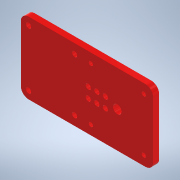
# Autodesk Inventor part: housingBack
Saved by Autodesk Inventor 2020 (Build 240168000, 168)
## iProperties
Created: 2020-02-03
Part Number: housingBack
Material: ABS Plastic
Document SubType Name: Modeling
Designer: Felix
Density: 1.06 g/cm^3
Appearance: Smooth - Red
Author: Felix
Autodesk Inventor part; units mm, degrees
ref_plane "YZ Plane" through (0, 0, 0) normal (1, 0, 0) x (0, 1, 0)
ref_plane "XZ Plane" through (0, 0, 0) normal (0, 1, 0) x (-1, 0, 0)
ref_plane "XY Plane" through (0, 0, 0) normal (0, 0, 1) x (1, 0, 0)
sketch "Sketch1" plane through (0, 0, 0) normal (0, 0, 1) x (1, 0, 0)
  line L0 (21.5, 21) -> (-21.5, 21) projected
  arc A0 (-21.5, 21) -> (-26, 16.5) centre (-21.5, 16.5) ccw construction
  line L1 (-26, 16.5) -> (-26, -16.5) construction
  arc A1 (-26, -16.5) -> (-21.5, -21) centre (-21.5, -16.5) ccw construction
  line L2 (-21.5, -21) -> (21.5, -21) projected
  arc A2 (21.5, -21) -> (26, -16.5) centre (21.5, -16.5) ccw construction
  line L3 (26, -16.5) -> (26, 16.5) construction
  arc A3 (26, 16.5) -> (21.5, 21) centre (21.5, 16.5) ccw construction
  circle A4 centre (5, 0) radius 2.5 projected
  circle A5 centre (-20, 15.5) radius 1.5 projected
  circle A6 centre (-10.5, -15.5) radius 1.2295 projected
  circle A7 centre (-10.5, 15.5) radius 1.2295 projected
  circle A8 centre (-2, 3) radius 1.5 projected
  circle A9 centre (-2, -3) radius 1.5 projected
  circle A10 centre (-7, 3) radius 1.5 projected
  circle A11 centre (-7, -3) radius 1.5 projected
  circle A12 centre (-12, 3) radius 1.5 projected
  circle A13 centre (-12, -3) radius 1.5 projected
  circle A14 centre (-20, -15.5) radius 1.5 projected
  circle A15 centre (20.5, -15.5) radius 1.2295 projected
  circle A16 centre (20.5, 15.5) radius 1.2295 projected
  line L4 (-21.5, 21) -> (-47, 21)
  line L5 (-51.5, 16.5) -> (-51.5, -16.5)
  line L6 (-47, -21) -> (-21.5, -21)
  arc A17 (-47, 21) -> (-51.5, 16.5) centre (-47, 16.5) ccw
  arc A18 (-51.5, -16.5) -> (-47, -21) centre (-47, -16.5) ccw
  circle A19 centre (-47, -16.5) radius 1.5
  circle A20 centre (-47, 16.5) radius 1.5
  line L7 (21.5, 21) -> (32, 21)
  line L8 (36.5, 16.5) -> (36.5, -16.5)
  line L9 (32, -21) -> (21.5, -21)
  arc A21 (36.5, 16.5) -> (32, 21) centre (32, 16.5) ccw
  arc A22 (32, -21) -> (36.5, -16.5) centre (32, -16.5) ccw
  circle A23 centre (32, 16.5) radius 1.5
  circle A24 centre (32, -16.5) radius 1.5
  point P0 (0, 0)
  point P1 (-51.5, 21)
  point P2 (36.5, 21)
  dimension "d0" = 30
  dimension "d1" = 4.5
  dimension "d2" = 3
  dimension "d3" = 3
  dimension "d13" = 15
  dimension "d14" = 4.5
  dimension "d15" = 3
  dimension "d16" = 3
  constraints: 12 end point, 9 point on circle, 8 centre point, 8 tangent, 5 point on line, 4 coincident, 3 perpendicular, 2 collinear, 2 equal radius, 1 horizontal
  measures "d0" distance of L0.end point (-51.5, 21)
  measures "d1" radius of A17
  measures "d2" diameter of A19
  measures "d3" diameter of A20
  measures "d13" distance of L7.start point (36.5, 21)
  measures "d14" radius of A21
  measures "d15" diameter of A23
  measures "d16" diameter of A24
extrude "Extrusion1" add sketch "Sketch1" along normal blind 3.5
ref_plane "Work Plane1" through (0, 0, 10.75) normal (0, 0, -1) x (-1, 0, 0)
sketch "Sketch2" plane through (0, 0, 0) normal (0, 0, -1) x (-1, 0, 0)
  circle A0 centre (-20.5, 15.5) radius 1.2295 projected
  circle A1 centre (-20.5, 15.5) radius 3
  circle A2 centre (10.5, 15.5) radius 1.2295 projected
  circle A3 centre (10.5, 15.5) radius 3
  circle A4 centre (-20.5, -15.5) radius 1.2295 projected
  circle A5 centre (-20.5, -15.5) radius 3
  circle A6 centre (10.5, -15.5) radius 1.2295 projected
  circle A7 centre (10.5, -15.5) radius 3
  point P0 (0, 0)
  dimension "d7" = 6
  dimension "d8" = 6
  dimension "d9" = 6
  dimension "d10" = 6
  constraints: 4 centre point, 4 coincident
  measures "d7" diameter of A1
  measures "d8" diameter of A3
  measures "d9" diameter of A5
  measures "d10" diameter of A7
extrude "Extrusion2" add sketch "Sketch2" along normal blind 3
equation "\"d7\" = d8"
equation "\"d9\" = d8"
equation "\"d10\" = d8"
body "Solid1"
